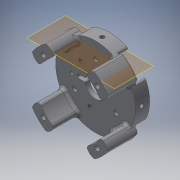
# Autodesk Inventor part: cycloid_outter_motor_fixer
Saved by Autodesk Inventor 2019.4 (Build 234330000, 330)
## iProperties
Created: 2019-09-11
Part Number: cycloid_outter_motor_fixer
Material: Generic
Document SubType Name: Modeling
Designer: cdi
Density: 1 g/cm^3
Appearance: Default
Author: cdi
Autodesk Inventor part; units mm, degrees
ref_plane "YZ Plane" through (0, 0, 0) normal (1, 0, 0) x (0, 1, 0)
ref_plane "XY Plane" through (0, 0, 0) normal (0, 0, 1) x (1, 0, 0)
sketch "Sketch1" plane through (0, 0, 0) normal (0, 0, 1) x (1, 0, 0)
  circle A0 centre (0, 0) radius 30
  circle A1 centre (0, 0) radius 23
  dimension "d0" = 60
  dimension "d1" = 7
  dimension "d27" = 46
  constraints: 2 centre point, 2 coincident
  measures "d0" diameter of A0
  measures "d1" radial gap between concentric circles of A0 A1
  measures "d27" diameter of A1
extrude "Extrusion1" add sketch "Sketch1" along normal blind 20
sketch "Sketch2" plane through (0, 0, 0) normal (0, 0, -1) x (-1, 0, 0)
  circle A0 centre (0, 0) radius 23 projected
extrude "Extrusion2" add sketch "Sketch2" against normal blind 3
sketch "Sketch3" plane through (0, 0, 0) normal (0, 0, -1) x (-1, 0, 0)
  line L0 (0, 0) -> (49.6899, 0)
  circle A0 centre (0, 0) radius 16
  circle A1 centre (11.3137, 11.3137) radius 1.5
  circle A2 centre (0, 0) radius 25.5
  line L1 (0, 0) -> (36.2318, 36.2318)
  circle A3 centre (18.0312, 18.0312) radius 1.5
  circle A4 centre (-15.4548, 4.1411) radius 1.5
  circle A5 centre (4.1411, -15.4548) radius 1.5
  circle A6 centre (-18.0312, 18.0312) radius 1.5
  circle A7 centre (-18.0312, -18.0312) radius 1.5
  circle A8 centre (18.0312, -18.0312) radius 1.5
  circle A9 centre (0, 16) radius 1.5
  circle A10 centre (-13.8564, -8) radius 1.5
  circle A11 centre (13.8564, -8) radius 1.5
  dimension "d9" = 51
  dimension "d6" = 32
  dimension "d8" = 3
  dimension "d10" = 45
  dimension "d11" = 3
  dimension "d14" = 360
  dimension "d18" = 360
  dimension "d118" = 3
  dimension "d121" = 360
  constraints: 11 centre point, 4 end point, 2 coincident, 2 point on circle, 2 point on line, 1 horizontal, 26 other
  measures "d6" diameter of A0
  measures "d8" diameter of A1
  measures "d10" angle of L0 L1
  measures "d11" diameter of A3
  measures "d118" diameter of A9
hole "Hole1" at (18.0312, 18.0312, 0) at (15.4548, 4.1411, 0) at (-18.0312, 18.0312, 0) at (-11.3137, 11.3137, 0) at (-4.1411, -15.4548, 0) at (18.0312, -18.0312, 0) at (-18.0312, -18.0312, 0) direction (0, 0, 1) diameter 3.3 end through all countersink diameter 6.5 countersink angle 90
sketch "Sketch4" plane through (0, 0, 0) normal (0, 0, -1) x (-1, 0, 0)
  circle A0 centre (-18.0312, 18.0312) radius 1.65 projected
  arc A1 (-10.8725, 20.2679) -> (-16.1394, 25.2887) centre (-18.0312, 18.0312) ccw
  circle A2 centre (0, 0) radius 30 projected
  circle A3 centre (0, 0) radius 23 projected
  circle A4 centre (18.0312, 18.0312) radius 1.65 projected
  arc A5 (16.1394, 25.2887) -> (10.8725, 20.2679) centre (18.0312, 18.0312) ccw
  arc A6 (16.1394, 25.2887) -> (-16.1394, 25.2887) centre (0, 0) ccw
  arc A7 (10.8725, 20.2679) -> (-10.8725, 20.2679) centre (0, 0) ccw
  point P0 (16.7006, 17.2363)
  point P1 (-16.7006, 17.2363)
  dimension "d28" = 15
  dimension "d29" = 15
  constraints: 10 point on circle, 4 centre point, 2 coincident, 1 concentric, 6 other
  measures "d28" diameter of A1
  measures "d29" diameter of A5
extrude "Extrusion3" cut sketch "Sketch4" against normal through all contours A1 A2 A5 A3 picked at (-6.3447, 26.7958)
pattern_circular "Circular Pattern1" count 4 over 360 about axis through (0, 0, 0) along (0, 0, 1) of "Extrusion3"
fillet "Fillet1" radius 1 4 edges at (-21.2132, 21.2132, 0) (21.2132, 21.2132, 0) (21.2132, -21.2132, 0) (-21.2132, -21.2132, 0)
fillet "Fillet2" radius 6 8 edges at (-10.8725, -20.2679, 1.5) (10.8725, -20.2679, 1.5) (20.2679, -10.8725, 1.5) (-20.2679, -10.8725, 1.5) (-20.2679, 10.8725, 1.5) (-10.8725, 20.2679, 1.5) (10.8725, 20.2679, 1.5) (20.2679, 10.8725, 1.5)
sketch "Sketch5" plane through (0, 0, 0) normal (0, 0, -1) x (-1, 0, 0)
  circle A0 centre (0, 0) radius 7
  dimension "d37" = 14
  constraints: 1 centre point, 1 coincident
  measures "d37" diameter of A0
extrude "Extrusion4" cut sketch "Sketch5" against normal through all
sketch "Sketch6" plane through (0, 0, 0) normal (0, 0, -1) x (-1, 0, 0)
  circle A0 centre (0, 0) radius 21
  circle A1 centre (-15.4548, 4.1411) radius 3.25 projected
  arc A2 (-20.804, 2.8621) -> (-19.4479, 7.9233) centre (-15.4548, 4.1411) ccw
  circle A3 centre (11.3137, 11.3137) radius 3.25 projected
  arc A4 (12.8807, 16.5858) -> (16.5858, 12.8807) centre (11.3137, 11.3137) ccw
  circle A5 centre (4.1411, -15.4548) radius 3.25 projected
  arc A6 (7.9233, -19.4479) -> (2.8621, -20.804) centre (4.1411, -15.4548) ccw
  dimension "d40" = 42
  dimension "d41" = 11
  dimension "d42" = 11
  dimension "d43" = 11
  constraints: 12 point on circle, 4 centre point, 4 coincident
  measures "d40" diameter of A0
  measures "d41" diameter of A4
  measures "d42" diameter of A2
  measures "d43" diameter of A6
extrude "Extrusion5" cut sketch "Sketch6" against normal blind 0.5 contours A0 A6 A2 A4
fillet "Fillet3" radius 2 6 edges at (19.4479, 7.9233, 0.25) (20.804, 2.8621, 0.25) (-12.8807, 16.5858, 0.25) (-16.5858, 12.8807, 0.25) (-2.8621, -20.804, 0.25) (-7.9233, -19.4479, 0.25)
sketch "Sketch7" plane through (0, 0, 0) normal (0, 0, -1) x (-1, 0, 0)
  arc A0 (12.7938, 23.3996) -> (-12.7938, 23.3996) centre (0, 0) ccw
  arc A1 (-12.7938, 23.3996) -> (-6.8238, 21.9644) centre (-8.6039, 27.6943) ccw projected
  arc A2 (6.8238, 21.9644) -> (-6.8238, 21.9644) centre (0, 0) ccw projected
  arc A3 (6.8238, 21.9644) -> (12.7938, 23.3996) centre (8.6039, 27.6943) ccw projected
  constraints: 4 point on circle, 1 centre point, 1 coincident
extrude "Extrusion6" add sketch "Sketch7" along normal blind 5
sketch "Sketch8" plane through (0, 0, -5) normal (0, 0, -1) x (-1, 0, 0)
  arc A0 (12.7938, 23.3996) -> (-12.7938, 23.3996) centre (0, 0) ccw projected
  arc A1 (11.431, 22.4021) -> (-11.431, 22.4021) centre (0, 0) ccw
  arc A2 (6.8238, 21.9644) -> (12.7938, 23.3996) centre (8.6039, 27.6943) ccw projected
  arc A3 (-12.7938, 23.3996) -> (-6.8238, 21.9644) centre (-8.6039, 27.6943) ccw projected
  dimension "d50" = 50.3
  constraints: 4 point on circle, 1 centre point, 1 coincident
  measures "d50" diameter of A1
extrude "Extrusion7" add sketch "Sketch8" along normal blind 1.6
sketch "Sketch9" plane through (0, 0, 0) normal (0, 0, 1) x (1, 0, 0)
  arc A0 (6.8238, 21.9644) -> (12.7938, 23.3996) centre (8.6039, 27.6943) ccw projected
  arc A1 (12.7938, 23.3996) -> (-12.7938, 23.3996) centre (0, 0) ccw projected
  arc A2 (-12.7938, 23.3996) -> (-6.8238, 21.9644) centre (-8.6039, 27.6943) ccw projected
  arc A3 (6.8238, 21.9644) -> (-6.8238, 21.9644) centre (0, 0) ccw projected
extrude "Extrusion8" add sketch "Sketch9" along normal up to surface (3 mm away)
sketch "Sketch10" plane through (0, 0, -5) normal (0, 0, -1) x (-1, 0, 0)
  circle A0 centre (0, 0) radius 24.5
  dimension "d55" = 49
  constraints: 1 centre point, 1 coincident
  measures "d55" diameter of A0
extrude "Extrusion9" cut sketch "Sketch10" against normal up to surface (5 mm away)
pattern_circular "Circular Pattern2" count 4 over 360 about axis through (0, 0, 0) along (0, 0, 1) of "Extrusion9", "Extrusion8", "Extrusion7", "Extrusion6"
fillet "Fillet5" radius 1 2 edges at (-12.7938, 23.3996, -3.3) (12.7938, 23.3996, -3.3)
pattern_circular "Circular Pattern3" count 4 over 360 about axis through (0, 0, 0) along (0, 0, 1) of "Fillet5"
sketch "Sketch11" plane through (0, 0, 0.5) normal (0, 0, -1) x (-1, 0, 0)
  circle A0 centre (16, 0) radius 1
  line L0 (0, 0) -> (38.1903, 0)
  circle A1 centre (16, 0) radius 2
  dimension "d66" = 2
  dimension "d67" = 16
  dimension "d68" = 4
  constraints: 2 centre point, 2 end point, 1 coincident, 1 horizontal, 1 point on line
  measures "d66" diameter of A0
  measures "d67" distance of L0.start A0.centre
  measures "d68" diameter of A1
extrude "Extrusion10" add sketch "Sketch11" along normal blind 4.5 contours L0 A1 A0 | A0 L0 A1
sketch "Sketch12" plane through (0, 0, 0.5) normal (0, 0, -1) x (-1, 0, 0)
  line L0 (6.4, -0.75) -> (12.4, -0.75)
  line L1 (12.4, -0.75) -> (12.4, 1.75)
  line L2 (12.4, 1.75) -> (6.4, 1.75)
  line L3 (6.4, 1.75) -> (6.4, -0.75)
  line L4 (6.4, -0.75) -> (12.4, 1.75) construction
  line L5 (12.4, -0.75) -> (6.4, 1.75) construction
  point P0 (0, 0)
  point P1 (9.4, 0.5)
  dimension "d72" = 9.4
  dimension "d73" = 6
  dimension "d74" = 2.5
  dimension "d75" = 0.5
  constraints: 12 end point, 2 midpoint, 2 parallel, 1 horizontal, 1 perpendicular
  measures "d72" horizontal distance of point (0, 0) point (9.4, 0.5)
  measures "d73" distance of L1.end L2.end
  measures "d74" distance of L0.end L1.end
  measures "d75" vertical distance of point (0, 0) point (9.4, 0.5)
extrude "Extrusion11" cut sketch "Sketch12" along normal blind 10 and the other way blind 10
fillet "Fillet7" radius 0.5 4 edges at (-12.4, -0.75, 1.75) (-12.4, 1.75, 1.75) (-6.7777, 1.75, 1.75) (-6.9597, -0.75, 1.75)
ref_plane "Work Plane1" through (0, 22, 0) normal (0, 1, 0) x (-1, 0, 0)
sketch "Sketch14" plane through (0, 22, 0) normal (0, 1, 0) x (-1, 0, 0)
  circle A0 centre (0, -1.5) radius 1.25
  point P0 (0, 0)
  dimension "d90" = 2.5
  dimension "d91" = 1.5
  constraints: 1 centre point
  measures "d90" diameter of A0
  measures "d91" distance of point (0, 0) A0.centre
extrude "Extrusion13" cut sketch "Sketch14" along normal blind 10
pattern_circular "Circular Pattern5" count 4 over 360 about axis through (0, 0, 0) along (0, 0, 1) of "Extrusion13"
sketch "Sketch15" plane through (0, 0, 0.5) normal (0, 0, -1) x (-1, 0, 0)
  arc A0 (7.3951, -0.75) -> (6.9021, -1.1667) centre (7.3951, -1.25) ccw projected
  arc A1 (6.6776, 2.1) -> (6.9021, -1.1667) centre (0, 0) ccw projected
  arc A2 (6.6776, 2.1) -> (7.1545, 1.75) centre (7.1545, 2.25) ccw projected
  line L0 (7.1545, 1.75) -> (11.9, 1.75) projected
  arc A3 (12.4, 1.25) -> (11.9, 1.75) centre (11.9, 1.25) ccw projected
  line L1 (12.4, 1.25) -> (12.4, -0.25) projected
  arc A4 (11.9, -0.75) -> (12.4, -0.25) centre (11.9, -0.25) ccw projected
  line L2 (11.9, -0.75) -> (7.3951, -0.75) projected
  arc A5 (9.6321, -15.1401) -> (12.8529, -16.6073) centre (11.6288, -15.0257) ccw projected
  arc A6 (12.8529, -16.6073) -> (19.4346, 7.9559) centre (0, 0) ccw projected
  arc A7 (19.4346, 7.9559) -> (15.9117, 8.2957) centre (17.5837, 7.1982) ccw projected
  arc A8 (8.2957, 15.9117) -> (15.9117, 8.2957) centre (11.3137, 11.3137) ccw projected
  arc A9 (8.2957, 15.9117) -> (7.9559, 19.4346) centre (7.1982, 17.5837) ccw projected
  arc A10 (7.9559, 19.4346) -> (-16.6073, 12.8529) centre (0, 0) ccw projected
  arc A11 (-16.6073, 12.8529) -> (-15.1401, 9.6321) centre (-15.0257, 11.6288) ccw projected
  arc A12 (-17.9278, -0.7716) -> (-15.1401, 9.6321) centre (-15.4548, 4.1411) ccw projected
  arc A13 (-17.9278, -0.7716) -> (-20.8088, -2.8273) centre (-18.827, -2.558) ccw projected
  arc A14 (-20.8088, -2.8273) -> (-2.8273, -20.8088) centre (0, 0) ccw projected
  arc A15 (-2.8273, -20.8088) -> (-0.7716, -17.9278) centre (-2.558, -18.827) ccw projected
  arc A16 (9.6321, -15.1401) -> (-0.7716, -17.9278) centre (4.1411, -15.4548) ccw projected
  circle A17 centre (16, 0) radius 2 projected
extrude "Extrusion14" add sketch "Sketch15" along normal up to surface (0.5 mm away)
sketch "Sketch17" plane through (-16, 0, 0.5) normal (0, 0, -1) x (-1, 0, 0)
  circle A0 centre (0, 0) radius 1 projected
  point P0 (-16, 0)
extrude "Extrusion16" cut sketch "Sketch17" against normal through all
sketch "Sketch18" plane through (0, 0, -6.6) normal (0, 0, -1) x (-1, 0, 0)
  line L0 (-12.5, -7.7355) -> (-12.5, -43.8722)
  line L1 (-12.5, -43.8722) -> (12.5, -43.8722)
  line L2 (12.5, -43.8722) -> (12.5, -7.7355)
  line L3 (12.5, -7.7355) -> (-12.5, -7.7355)
  line L4 (-12.5, -7.7355) -> (12.5, -43.8722) construction
  line L5 (-12.5, -43.8722) -> (12.5, -7.7355) construction
  point P0 (0, 0)
  point P1 (0, -25.8039)
  dimension "d110" = 25
  constraints: 12 end point, 2 midpoint, 2 parallel, 1 perpendicular, 1 vertical
  measures "d110" distance of L1.end L0.end
extrude "Extrusion17" cut sketch "Sketch18" against normal up to surface (6.6 mm away)
fillet "Fillet13" radius 2 6 edges at (-11.6384, 21.9532, 3) (-16.2635, 16.2635, 3) (-12.7938, 23.3996, 1.5) (-21.9532, 11.6384, 3) (-20.2679, 10.8725, 11.5) (-10.8725, 20.2679, 11.5)
pattern_circular "Circular Pattern7" count 4 over 360 about axis through (0, 0, 0) along (0, 0, -1) of "Fillet13"
fillet "Fillet14" radius 2 1 edges at (-14, 0, 0)
sketch "Sketch19" plane through (0, 0, 0) normal (0, 0, -1) x (-1, 0, 0)
  circle A0 centre (0, 0) radius 16
  circle A1 centre (0, 16) radius 1.5
  circle A2 centre (-13.8564, -8) radius 1.5
  circle A3 centre (13.8564, -8) radius 1.5
  dimension "d123" = 32
  dimension "d124" = 3
  dimension "d134" = 360
  constraints: 3 centre point, 1 coincident, 1 vertical alignment, 9 other
  measures "d124" diameter of A1
hole "Hole2" at (13.8564, -8, 0) at (-13.8564, -8, 0) at (0, 16, 0) direction (0, 0, 1) diameter 3.2 end through all countersink diameter 6.5 countersink angle 90
sketch "Sketch22" plane through (0, 0, 0) normal (0, 0, -1) x (-1, 0, 0)
  circle A0 centre (-15.4548, 4.1411) radius 1.65 projected
  circle A1 centre (-15.4548, 4.1411) radius 4.7152
  circle A2 centre (11.3137, 11.3137) radius 1.65 projected
  circle A3 centre (11.3137, 11.3137) radius 4.6095
  circle A4 centre (4.1411, -15.4548) radius 1.65 projected
  circle A5 centre (4.1411, -15.4548) radius 4.6407
  point P0 (0, 0)
  constraints: 3 centre point, 3 coincident
extrude "Extrusion18" add sketch "Sketch22" against normal up to surface (3 mm away) contours A0 | A1 | A2 | A3 | A4 | A5
sketch "Sketch23" plane through (0, 0, 0) normal (0, 0, -1) x (-1, 0, 0)
  circle A0 centre (0, 0) radius 14
  circle A1 centre (9.8995, 9.8995) radius 1.5
  line L0 (9.8995, 9.8995) -> (0, 0)
  line L1 (0, 0) -> (21.6121, 0)
  dimension "d164" = 28
  dimension "d165" = 3
  dimension "d166" = 45
  constraints: 4 end point, 1 centre point, 1 coincident, 1 horizontal, 3 other
  measures "d165" diameter of A1
  measures "d166" angle of L0 L1
hole "Hole5" at (-9.8995, 9.8995, 0) direction (0, 0, 1) diameter 2.85 end through all thread size "M3.5x0.6" class "6H" standard "ISO Metric profile"
pattern_circular "Circular Pattern8" count 3 over 360 about axis through (0, 0, 0) along (0, 0, 1) of "Hole5"
chamfer "Chamfer1" distance 0.5 angle 45 3 edges at (12.2889, 4.336, 0) (-9.8995, 8.4745, 0) (-2.3894, -12.8105, 0)
chamfer "Chamfer2" distance 0.2 angle 45 4 edges at (1.25, 26.6394, -1.4958) (-26.6394, 1.25, -1.4958) (26.6394, -1.25, -1.4958) (-15, 0, -4)
body "Solid1"
